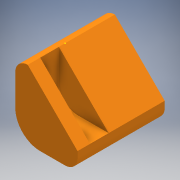
# Autodesk Inventor part: Plate Adapter
Saved by Autodesk Inventor 2017 (Build 210142000, 142)
## iProperties
Created: 2017-04-02
Part Number: Plate Adapter
Material: Generic
Document SubType Name: Modeling
Designer: gilef
Density: 1 g/cm^3
Appearance: Orange
Author: gilef
Autodesk Inventor part; units mm, degrees
ref_plane "YZ Plane" through (0, 0, 0) normal (1, 0, 0) x (0, 1, 0)
ref_plane "XZ Plane" through (0, 0, 0) normal (0, 1, 0) x (-1, 0, 0)
ref_plane "XY Plane" through (0, 0, 0) normal (0, 0, 1) x (1, 0, 0)
sketch "Sketch1" plane through (0, 0, 0) normal (0, 1, 0) x (-1, 0, 0)
  line L0 (0, 0) -> (0, -5)
  arc A0 (-3, -8) -> (0, -5) centre (-3, -5) ccw
  line L1 (-3, -8) -> (-8, -8)
  line L2 (-8, -8) -> (0, 0)
  line L3 (0, 0) -> (2, 0)
  line L4 (2, 0) -> (2, -7)
  arc A1 (-2, -11) -> (2, -7) centre (-2, -7) ccw
  line L5 (-8, -11) -> (-2, -11)
  line L6 (-8, -11) -> (-8, -8)
  dimension "d0" = 5
  dimension "d1" = 3
  dimension "d2" = 4
  dimension "d3" = 3
  dimension "d11" = 2
  constraints: 14 end point, 4 point on circle, 4 tangent, 3 horizontal, 3 vertical, 2 centre point, 1 perpendicular
  measures "d0" distance of L0.start L0.end
  measures "d1" radius of A0
  measures "d2" radius of A1
  measures "d3" distance of L5.start L1.end
  measures "d11" distance of L0.start L3.end
extrude "Extrusion1" add sketch "Sketch1" along normal blind 6 contours L3 L4 A1 L5 L6 L1 A0 L0
sketch "Sketch2" plane through (0, 6, 0) normal (0, 1, 0) x (1, 0, 0)
  line L0 (0, 0) -> (0, 5) projected
  arc A0 (3, 8) -> (0, 5) centre (3, 5) ccw projected
  line L1 (3, 8) -> (8, 8) projected
  line L2 (0, 0) -> (8, 8)
  line L3 (0, 0) -> (0, 5)
  line L4 (8, 8) -> (3, 8)
  arc A1 (3, 8) -> (0, 5) centre (3, 5) ccw
  constraints: 6 end point, 4 point on circle, 1 centre point, 1 horizontal, 1 tangent, 1 vertical
extrude "Extrusion2" add sketch "Sketch2" against normal blind 1
sketch "Sketch3" plane through (0, 0, 0) normal (0, -1, 0) x (1, 0, 0)
  line L0 (0, 0) -> (0, -5) projected
  arc A0 (0, -5) -> (3, -8) centre (3, -5) ccw projected
  line L1 (3, -8) -> (8, -8) projected
  line L2 (8, -8) -> (0, 0) projected
  line L3 (0, 0) -> (8, -8)
  line L4 (8, -8) -> (3, -8)
  line L5 (0, 0) -> (0, -5)
  arc A1 (0, -5) -> (3, -8) centre (3, -5) ccw projected
  arc A2 (0, -5) -> (0, -5) centre (5.2399, -2.7601) ccw
  arc A3 (0, -5) -> (3, -8) centre (3, -5) ccw
  constraints: 6 end point, 2 collinear, 2 point on circle, 1 centre point, 1 tangent, 1 vertical, 4 other
extrude "Extrusion3" add sketch "Sketch3" against normal blind 2 contours L2 A2 L0 | A2 L2 L1 L0 | A2 A0 | L2 L1 A2
fillet "Fillet1" radius 2 2 edges at (-2, 3, 0) (8, 3, -11)
sketch "Sketch4" plane through (0, 6, 0) normal (0, 1, 0) x (1, 0, 0)
  point P0 (0, 0)
sketch "Sketch5" plane through (0, 6, 0) normal (0, 1, 0) x (1, 0, 0)
  circle A0 centre (2, 7) radius 1.5
  line L0 (6, 11) -> (2, 11) projected
  line L1 (-2, 7) -> (-2, 2) projected
  point P0 (0, 0)
  dimension "d12" = 3
  dimension "d13" = 2.5
  dimension "d14" = 2.5
  constraints: 1 centre point
  measures "d12" diameter of A0
  measures "d13" distance edge to line of A0 L0
  measures "d14" distance edge to line of A0 L1
sketch "Sketch7" plane through (0, 6, 0) normal (0, 1, 0) x (1, 0, 0)
  arc A0 (2, 11) -> (-2, 7) centre (2, 7) ccw projected
  line L0 (-0.2454, 9.2454) -> (2.8219, 10.0672)
  line L1 (2.8219, 10.0672) -> (5.0672, 7.8219)
  line L2 (5.0672, 7.8219) -> (4.2454, 4.7546)
  line L3 (4.2454, 4.7546) -> (1.1781, 3.9328)
  line L4 (1.1781, 3.9328) -> (-1.0672, 6.1781)
  line L5 (-1.0672, 6.1781) -> (-0.2454, 9.2454)
  arc A1 (2, 11) -> (-2, 7) centre (2, 7) ccw projected
  line L6 (0, 0) -> (8, 8) projected
  line L7 (-1.0672, 6.1781) -> (-1.9985, 7.1094)
  line L8 (2.8219, 10.0672) -> (1.8906, 10.9985)
  line L9 (-2, 7) -> (-2, 2) projected
  line L10 (-2, 2) -> (-2, 7)
  arc A2 (-1.9985, 7.1094) -> (-2, 7) centre (2, 7) ccw
  line L11 (6, 11) -> (2, 11) projected
  line L12 (6, 11) -> (2, 11)
  arc A3 (2, 11) -> (1.8906, 10.9985) centre (2, 7) ccw
  line L13 (6, 11) -> (2, 11) projected
  arc A4 (-2, 2) -> (0, 0) centre (0, 2) ccw projected
  line L14 (8, 8) -> (8, 9) projected
  arc A5 (8, 9) -> (6, 11) centre (6, 9) ccw projected
  line L15 (8, 8) -> (0, 0) projected
  arc A6 (-2, 2) -> (0, 0) centre (0, 2) ccw
  line L16 (-2, 7) -> (-2, 2) projected
  line L17 (0, 0) -> (8, 8)
  line L18 (8, 9) -> (8, 8)
  arc A7 (8, 9) -> (6, 11) centre (6, 9) ccw projected
  arc A8 (8, 9) -> (6, 11) centre (6, 9) ccw
  dimension "d15" = 5.5
  constraints: 24 end point, 12 point on circle, 5 collinear, 4 centre point, 4 tangent, 2 coincident, 1 parallel, 1 perpendicular, 13 other
  measures "d15" distance between parallel lines of L1 L4
extrude "Extrusion4" add sketch "Sketch7" along normal blind 6 contours L11 A5 L14 L6 A4 L9 A0 L7 L4 L3 L2 L1 L8
sketch "Sketch8" plane through (0, 12, 0) normal (0, 1, 0) x (1, 0, 0)
  line L0 (4.2454, 4.7546) -> (1.1781, 3.9328) projected
  line L1 (1.1781, 3.9328) -> (-1.9985, 7.1094) projected
  line L2 (5.0672, 7.8219) -> (4.2454, 4.7546) projected
  line L3 (1.8906, 10.9985) -> (5.0672, 7.8219) projected
  line L4 (4.2454, 4.7546) -> (1.1781, 3.9328)
  line L5 (1.1781, 3.9328) -> (-1.0672, 6.1781)
  line L6 (-1.0672, 6.1781) -> (-0.2454, 9.2454)
  line L7 (-0.2454, 9.2454) -> (2.8219, 10.0672)
  line L8 (2.8219, 10.0672) -> (5.0672, 7.8219)
  line L9 (5.0672, 7.8219) -> (4.2454, 4.7546)
  arc A0 (1.8906, 10.9985) -> (-1.9985, 7.1094) centre (2, 7) ccw projected
  line L10 (-1.0672, 6.1781) -> (-1.9985, 7.1094)
  line L11 (2.8219, 10.0672) -> (1.8906, 10.9985)
  arc A1 (1.8906, 10.9985) -> (-1.9985, 7.1094) centre (2, 7) ccw
  point P0 (0, 0)
  point P1 (2, 7)
  point P2 (2, 7)
  constraints: 16 end point, 2 point on circle, 1 centre point, 1 coincident, 1 collinear, 1 concentric, 13 other
extrude "Extrusion5" add sketch "Sketch8" against normal blind 2 contours L1 A0 L3 L7 L6
sketch "Sketch9" plane through (0, 12, 0) normal (0, 1, 0) x (1, 0, 0)
  line L0 (2.8219, 10.0672) -> (5.0672, 7.8219) projected
  line L1 (5.0672, 7.8219) -> (4.2454, 4.7546) projected
  line L2 (4.2454, 4.7546) -> (1.1781, 3.9328) projected
  line L3 (1.1781, 3.9328) -> (-1.0672, 6.1781) projected
  line L4 (-1.0672, 6.1781) -> (-0.2454, 9.2454) projected
  line L5 (-0.2454, 9.2454) -> (2.8219, 10.0672) projected
  arc A0 (2, 11) -> (-2, 7) centre (2, 7) ccw projected
  line L6 (-2, 7) -> (-2, 2) projected
  arc A1 (-2, 2) -> (0, 0) centre (0, 2) ccw projected
  line L7 (0, 0) -> (8, 8) projected
  line L8 (8, 8) -> (8, 9) projected
  arc A2 (8, 9) -> (6, 11) centre (6, 9) ccw projected
  line L9 (6, 11) -> (2, 11) projected
  point P0 (0, 0)
extrude "Extrusion6" add sketch "Sketch9" along normal blind 2 contours L0 L1 L2 L3 L4 L5 | L9 A2 L8 L7 A1 L6 A0
extrude "Extrusion7" cut sketch "Sketch5" along normal through all
body "Solid1"
